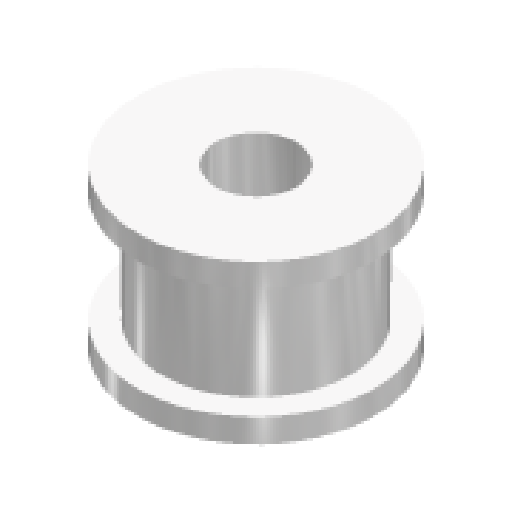
# Autodesk Inventor part: 6mm toothed idler
Saved by Autodesk Inventor 2023.2 (Build 272271000, 271)
## iProperties
Created: 2023-02-03
Part Number: 6mm toothed idler
Material: Aluminum 6061
Document SubType Name: Modeling
Designer: remop
Density: 2.7 g/cm^3
Appearance: Aluminum - Polished
Author: remop
Autodesk Inventor part; units mm, degrees
ref_plane "YZ Plane" through (0, 0, 0) normal (1, 0, 0) x (0, 1, 0)
ref_plane "XZ Plane" through (0, 0, 0) normal (0, 1, 0) x (-1, 0, 0)
ref_plane "XY Plane" through (0, 0, 0) normal (0, 0, 1) x (1, 0, 0)
sketch "Sketch1" plane through (0, 0, 0) normal (1, 0, 0) x (0, 1, 0)
  line L0 (0, 0) -> (17.2785, 0)
  line L1 (0, -2.5) -> (10, -2.5)
  line L2 (10, -2.5) -> (10, -7.5)
  line L3 (10, -7.5) -> (8.5, -7.5)
  line L4 (8.5, -7.5) -> (8.5, -6)
  line L5 (8.5, -6) -> (1.5, -6)
  line L6 (1.5, -6) -> (1.5, -7.5)
  line L7 (1.5, -7.5) -> (0, -7.5)
  line L8 (0, -7.5) -> (0, -2.5)
  point P0 (5, -2.5)
  dimension "d1" = 5
  dimension "d2" = 15
  dimension "d3" = 12
  dimension "d4" = 7
  dimension "d5" = 1.5
  constraints: 18 end point, 6 perpendicular, 2 horizontal, 2 point on line, 1 collinear, 1 midpoint, 1 vertical alignment, 1 other
  measures "d1" diameter of L1 L0
  measures "d2" diameter of L7 L0
  measures "d3" diameter of L5 L0
  measures "d4" distance of L4.end L5.end
  measures "d5" distance of L6.end L7.end
revolve "Revolution1" add sketch "Sketch1" angle 360 about axis through (0, 0, 0) along (0, 1, 0)
body "Solid1"
